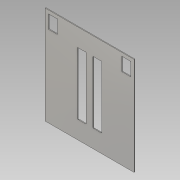
# Autodesk Inventor part: Interior Frame
Saved by Autodesk Inventor 2016 (Build 200138000, 138)
## iProperties
Created: 2017-05-19
Part Number: Interior Frame
Material: Generic
Document SubType Name: Modeling
Designer: 31745
Density: 1 g/cm^3
Appearance: Default
Author: 31745
Autodesk Inventor part; units mm, degrees
ref_plane "YZ Plane" through (0, 0, 0) normal (1, 0, 0) x (0, 1, 0)
ref_plane "XZ Plane" through (0, 0, 0) normal (0, 1, 0) x (-1, 0, 0)
ref_plane "XY Plane" through (0, 0, 0) normal (0, 0, 1) x (1, 0, 0)
sketch "Sketch1" plane through (0, 0, 0) normal (0, 0, 1) x (1, 0, 0)
  line L0 (0, 0) -> (254, 0)
  line L1 (254, 0) -> (254, 279.4)
  line L2 (254, 279.4) -> (0, 279.4)
  line L3 (0, 279.4) -> (0, 0)
  line L4 (92.075, 228.6) -> (117.475, 228.6)
  line L5 (117.475, 228.6) -> (117.475, 50.8)
  line L6 (117.475, 50.8) -> (92.075, 50.8)
  line L7 (92.075, 50.8) -> (92.075, 228.6)
  line L8 (136.525, 228.6) -> (161.925, 228.6)
  line L9 (161.925, 228.6) -> (161.925, 50.8)
  line L10 (161.925, 50.8) -> (136.525, 50.8)
  line L11 (136.525, 50.8) -> (136.525, 228.6)
  line L12 (117.475, 228.6) -> (136.525, 228.6)
  point P0 (127, 228.6)
  point P1 (127, 279.4)
  dimension "d0" = 254
  dimension "d1" = 279.4
  dimension "d2" = 19.05
  dimension "d3" = 25.4
  dimension "d4" = 25.4
  dimension "d5" = 50.8
  dimension "d6" = 50.8
  constraints: 26 end point, 6 parallel, 4 horizontal, 3 perpendicular, 2 midpoint, 2 point on line, 1 vertical alignment
  measures "d0" distance of L2.end L1.end
  measures "d1" distance of L1.end L0.end
  measures "d2" distance of L4.end L8.start
  measures "d3" distance of L8.start L8.end
  measures "d4" distance of L4.start L4.end
  measures "d5" distance between parallel lines of L2 L8
  measures "d6" distance between parallel lines of L0 L10
extrude "Extrusion1" add sketch "Sketch1" along normal blind 2.286
fillet "Fillet1" radius 1.5875 8 edges at (92.075, 50.8, 1.143) (117.475, 50.8, 1.143) (136.525, 50.8, 1.143) (161.925, 50.8, 1.143) (161.925, 228.6, 1.143) (136.525, 228.6, 1.143) (117.475, 228.6, 1.143) (92.075, 228.6, 1.143)
sketch "Sketch2" plane through (0, 0, 2.286) normal (0, 0, 1) x (1, 0, 0)
  line L0 (9.525, 269.875) -> (34.925, 269.875)
  line L1 (34.925, 269.875) -> (34.925, 231.775)
  line L2 (34.925, 231.775) -> (9.525, 231.775)
  line L3 (9.525, 231.775) -> (9.525, 269.875)
  line L4 (219.075, 269.875) -> (244.475, 269.875)
  line L5 (244.475, 269.875) -> (244.475, 231.775)
  line L6 (244.475, 231.775) -> (219.075, 231.775)
  line L7 (219.075, 231.775) -> (219.075, 269.875)
  line L8 (0, 279.4) -> (0, 0) projected
  line L9 (254, 0) -> (254, 279.4) projected
  line L10 (254, 279.4) -> (0, 279.4) projected
  dimension "d10" = 9.525
  dimension "d11" = 9.525
  dimension "d12" = 9.525
  dimension "d13" = 25.4
  dimension "d14" = 38.1
  constraints: 16 end point, 4 parallel, 2 horizontal, 2 horizontal alignment, 2 perpendicular, 1 collinear
  measures "d10" distance between parallel lines of L8 L3
  measures "d11" distance between parallel lines of L9 L5
  measures "d12" distance between parallel lines of L10 L4
  measures "d13" distance of L0.start L0.end
  measures "d14" distance of L0.end L1.end
extrude "Extrusion2" cut sketch "Sketch2" against normal through all
equation "\"d4\" = d3"
equation "\"d11\" = d10"
body "Solid1"
